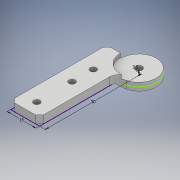
# Autodesk Inventor part: revHinge2
Saved by Autodesk Inventor 2018.2 (Build 222227000, 227)
## iProperties
Created: 2018-03-30
Part Number: revHinge2
Material: Generic
Document SubType Name: Modeling
Designer: mzhang
Density: 1 g/cm^3
Appearance: Default
Author: mzhang
Autodesk Inventor part; units mm, degrees
ref_plane "YZ Plane" through (0, 0, 0) normal (1, 0, 0) x (0, 1, 0)
ref_plane "XZ Plane" through (0, 0, 0) normal (0, 1, 0) x (-1, 0, 0)
ref_plane "XY Plane" through (0, 0, 0) normal (0, 0, 1) x (1, 0, 0)
sketch "Sketch1" plane through (0, 0, 0) normal (0, 0, 1) x (1, 0, 0)
  line L0 (0, 0) -> (15, 0)
  line L1 (15, 0) -> (15, -50)
  line L2 (15, -50) -> (0, -50)
  line L3 (0, -50) -> (0, 0)
  circle A0 centre (16.75, 0) radius 1.75
  circle A1 centre (16.75, 0) radius 9.0322
  dimension "d12" = 3.5
  dimension "d0" = 15
  dimension "d1" = 50
  constraints: 8 end point, 2 parallel, 1 centre point, 1 coincident, 1 horizontal, 1 horizontal alignment, 1 perpendicular, 2 other
  measures "d0" distance of L1.end L2.end
  measures "d1" distance of L0.end L1.end
extrude "Extrusion1" add sketch "Sketch1" along normal blind 4 contours L0 A1 L1 L2 L3 | L0 L1 A1 picked at (14.3439, -5.6975)
chamfer "Chamfer2" distance 2 angle 45 1 edges at (0, 0, 2)
sketch "Sketch2" plane through (0, 0, 4) normal (0, 0, 1) x (1, 0, 0)
  circle A0 centre (7.5, -43.8644) radius 1.625
  circle A1 centre (7.5, -14.4752) radius 1.625
  point P0 (0, 0)
  dimension "d10" = 3.25
  dimension "d11" = 3.25
  constraints: 2 centre point
  measures "d10" diameter of A0
  measures "d11" diameter of A1
extrude "Extrusion2" cut sketch "Sketch2" against normal up to surface (4 mm away)
extrude "Extrusion3" add sketch "Sketch1" along normal mid plane 4 contours A1 L1 L0 | L0 L1 A1
chamfer "Chamfer3" distance 2 angle 45 1 edges at (9.7719, -5.7348, 0)
sketch "Sketch3" plane through (0, 0, 4) normal (0, 0, 1) x (1, 0, 0)
  circle A0 centre (16.75, 0) radius 9.0322 projected
  circle A1 centre (16.75, 0) radius 9.5322
  point P0 (0, 0)
  dimension "d20" = 0.5
  constraints: 1 centre point
  measures "d20" radial gap between concentric circles of A0 A1
extrude "Extrusion4" cut sketch "Sketch3" against normal up to surface (2 mm away) contours A0 | A1
fillet "Fillet1" radius 5 1 edges at (15, -8.8611, 0)
chamfer "Chamfer4" distance 2 angle 45 2 edges at (0, -50, 2) (15, -50, 2)
sketch "Sketch4" plane through (0, 0, 4) normal (0, 0, 1) x (1, 0, 0)
  circle A0 centre (7.5, -25.5328) radius 1.625
  point P0 (0, 0)
  dimension "d27" = 3.25
  constraints: 1 centre point
  measures "d27" diameter of A0
extrude "Extrusion5" cut sketch "Sketch4" against normal up to surface (4 mm away)
body "Solid1"
